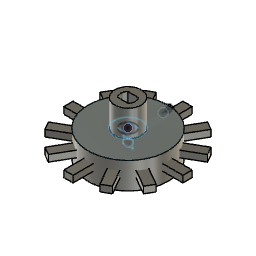
Tank Track Gear v1 (Autodesk Fusion 360 design; units mm, degrees)
Autodesk Fusion 360 part; units mm, degrees
sketch "Sketch1" plane through (0, 0, 0) normal (0, 0, 1) x (1, 0, 0)
  circle A0 centre (0, 0) radius 15
  dimension "d1" = 30
  constraint coincident A0.centre origin
  measures "d1" diameter of A0
extrude "Extrude1" add sketch "Sketch1" along normal blind 10 makes body 1
sketch "Sketch2" plane through (0, 0, 0) normal (0, 1, 0) x (1, 0, 0)
  line L0 (-1.75, -4.1374) -> (1.75, -4.1374)
  line L1 (1.75, -4.1374) -> (1.75, -6.6374)
  line L2 (1.75, -6.6374) -> (-1.75, -6.6374)
  line L3 (-1.75, -6.6374) -> (-1.75, -4.1374)
  line L4 (-1.75, -4.1374) -> (1.75, -6.6374) construction
  line L5 (1.75, -4.1374) -> (-1.75, -6.6374) construction
  point P0 (0, -5.3874)
  dimension "d4" = 2.5
  dimension "d5" = 3.5
  constraint horizontal L0
  constraint perpendicular L0 L1
  constraint parallel L0 L2
  constraint parallel L1 L3
  constraint coincident L4 P0
  constraint coincident L5 P0
  measures "d4" distance of L0.start L2.end
  measures "d5" distance of L0.start L0.end
extrude "Extrude3" add sketch "Sketch2" along normal blind 36 separate body makes body 2
extrude "Extrude4" cut 1 faces at (0.5833, 36, 4.9708) along direction (0, -1, 0) blind 18 on bodies 2 bodies 2
extrude "Extrude5" cut 1 faces at (0.5833, 18, 4.9708) along direction (0, -1, 0) blind 1 on bodies 2 bodies 2
sketch "Sketch6" plane through (-1.75, 0, 0) normal (-1, 0, 0) x (0, -1, 0)
  line L0 (-17, 6.6374) -> (-17, 4.1374)
  line L1 (-17, 4.1374) -> (0, 4.1374)
  line L2 (0, 4.1374) -> (0, 6.6374)
  line L3 (0, 6.6374) -> (-17, 6.6374)
  line L4 (-17, 6.6374) -> (-15, 6.6374)
  constraint coincident L0.start L3.end
  constraint coincident L3 L4.end
  constraint perpendicular L0 L4
extrude "Extrude6" add 1 faces at (0.5833, 17, 4.9708) along direction (0, 1, 0) blind 0.5 on bodies 2 bodies 2
extrude "Extrude22" add 1 faces at (0.5833, 17.5, 4.9708) along direction (0, 1, 0) blind 5 on bodies 2 bodies 2
pattern_circular "C-Pattern1" count 12 over 360 about axis through (0, 0, 0) along (0, 0, 1) of bodies 2 makes body 3 at (-6.9948, 13.282, 4.1374) makes body 4 at (-6.7869, 3.2448, 4.1374) makes body 5 at (-7.5, 0.5833, 6.6374) makes body 6 at (-13.282, -6.9948, 4.1374) makes body 7 at (-8.0052, -12.6987, 4.1374) makes body 8 at (0.5833, -7.5, 4.1374) makes body 9 at (8.0052, -12.6987, 6.6374) makes body 10 at (6.2035, -4.2552, 6.6374) makes body 11 at (7.5, -0.5833, 6.6374) makes body 12 at (13.282, 6.9948, 4.1374) makes body 13 at (3.2448, 6.7869, 4.1374)
sketch "Sketch9" plane through (0, 0, 10) normal (0, 0, 1) x (-1, 0, 0)
  circle A0 centre (0, 0) radius 15
  circle A1 centre (0, 0) radius 2.75
  line L0 (-1.9765, 1.9121) -> (1.9765, 1.9121)
  line L1 (-1.9765, -1.9121) -> (1.9765, -1.9121)
  circle A2 centre (0, 0) radius 5
  dimension "d61" = 5.5
  constraint coincident A0.centre A1.centre
  constraint coincident A1 L0.start
  constraint coincident A1 L0.end
  constraint horizontal L0
  constraint coincident A1 L1.start
  constraint coincident A1 L1.end
  constraint parallel L0 L1
  measures "d61" diameter of A1
extrude "Extrude23" add sketch "Sketch9" along normal blind 10 contours A1 L0 | A1 L1 | A2 bodies 1
extrude "Extrude21" [suppressed]
